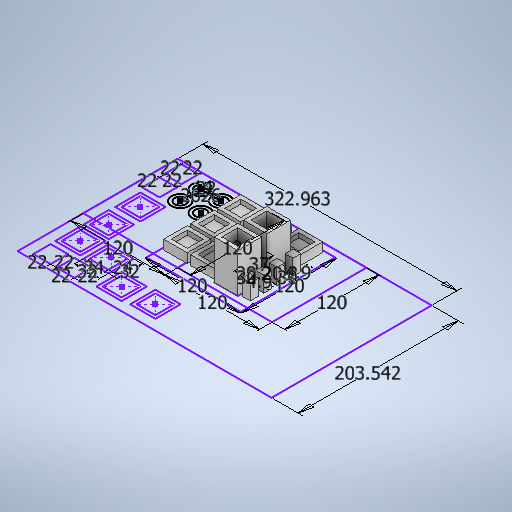
# Autodesk Inventor part: axie1
Saved by Autodesk Inventor 2025.1 (Build 291241000, 241)
## iProperties
Created: 2024-10-25
Part Number: axie1
Material: 一般
Document SubType Name: Modeling
Designer: youtian
Density: 1 g/cm^3
Appearance: 預設
Author: youtian
Autodesk Inventor part; units mm, degrees
ref_plane "YZ Plane" through (0, 0, 0) normal (1, 0, 0) x (0, 1, 0)
ref_plane "XZ Plane" through (0, 0, 0) normal (0, 1, 0) x (-1, 0, 0)
ref_plane "XY Plane" through (0, 0, 0) normal (0, 0, 1) x (1, 0, 0)
sketch "草圖1" plane through (0, 0, 0) normal (0, 1, 0) x (-1, 0, 0)
  circle A0 centre (0, 0) radius 7
  circle A1 centre (0, 0) radius 11
  line L0 (0, 0) -> (-26.517, 0)
  line L1 (0, 0) -> (0, 28.4195)
  circle A2 centre (-26, 0) radius 7
  circle A3 centre (-26, 0) radius 11
  circle A4 centre (0, 26) radius 7
  circle A5 centre (0, 26) radius 11
  circle A6 centre (-26, 26) radius 7
  circle A7 centre (-26, 26) radius 11
  dimension "d0" = 14
  dimension "d1" = 22
  dimension "d6" = 26
  dimension "d9" = 26
  constraints: 8 centre point, 5 coincident, 4 end point, 2 horizontal, 2 vertical, 12 other
  measures "d0" diameter of A0
  measures "d1" diameter of A1
  measures "d6" distance of A0.centre A2.centre
  measures "d9" distance of A0.centre A4.centre
sketch "草圖2" plane through (0, 0, 0) normal (0, 1, 0) x (-1, 0, 0)
  line L0 (-43.4184, -7.5692) -> (-73.4184, -7.5692)
  line L1 (-73.4184, -7.5692) -> (-73.4184, 22.4308)
  line L2 (-73.4184, 22.4308) -> (-43.4184, 22.4308)
  line L3 (-43.4184, 22.4308) -> (-43.4184, -7.5692)
  point P0 (0, 0)
  dimension "d14" = 30
  dimension "d15" = 30
  constraints: 8 end point, 2 parallel, 1 horizontal, 1 perpendicular
  measures "d14" distance of L1.end L2.end
  measures "d15" distance of L0.end L1.end
extrude "擠出3" add sketch "草圖2" along normal blind 12
sketch "草圖3" plane through (0, 12, 0) normal (0, 1, 0) x (1, 0, 0)
  line L0 (73.4184, -22.4308) -> (73.4184, 7.5692) projected
  line L1 (73.4184, 7.5692) -> (41.0142, -24.4308)
  line L2 (73.4184, 7.5692) -> (43.4184, 7.5692) projected
  line L3 (43.4184, 7.5692) -> (73.4184, -22.4308)
  line L4 (48.3184, 2.6692) -> (68.5184, 2.6692)
  line L5 (68.5184, 2.6692) -> (68.5184, -17.5308)
  line L6 (68.5184, -17.5308) -> (48.3184, -17.5308)
  line L7 (48.3184, -17.5308) -> (48.3184, 2.6692)
  line L8 (48.3184, 2.6692) -> (68.5184, -17.5308) construction
  line L9 (68.5184, 2.6692) -> (48.3184, -17.5308) construction
  point P0 (0, 0)
  point P1 (58.4184, -7.4308)
  dimension "d18" = 20.2
  dimension "d19" = 20.2
  constraints: 16 end point, 3 midpoint, 2 parallel, 1 horizontal, 1 perpendicular
  measures "d18" distance of L5.end L6.end
  measures "d19" distance of L4.end L5.end
extrude "擠出4" cut sketch "草圖3" against normal blind 5.6 contours L6 L7 L1 L3 | L3 L1 L4 L5 | L1 L3 L4 | L1 L7 L3
pattern_linear "矩形陣列1" count 2 spacing 34 along (1, 0, 0) count 3 spacing 34 along (0, 0, 1) of "擠出3", "擠出4"
sketch "草圖6" plane through (0, 0, 0) normal (0, 1, 0) x (-1, 0, 0)
  point P0 (0, 0)
sketch "草圖9" plane through (0, 0, 0) normal (0, 1, 0) x (-1, 0, 0)
  line L0 (-111.1142, 26.8484) -> (-141.1142, 26.8484)
  line L1 (-141.1142, 26.8484) -> (-141.1142, 56.8484)
  line L2 (-141.1142, 56.8484) -> (-111.1142, 56.8484)
  line L3 (-111.1142, 56.8484) -> (-111.1142, 26.8484)
  line L4 (-116.0142, 31.7484) -> (-136.2142, 31.7484)
  line L5 (-136.2142, 31.7484) -> (-136.2142, 51.9484)
  line L6 (-136.2142, 51.9484) -> (-116.0142, 51.9484)
  line L7 (-116.0142, 51.9484) -> (-116.0142, 31.7484)
  line L8 (-116.0142, 31.7484) -> (-136.2142, 51.9484) construction
  line L9 (-136.2142, 31.7484) -> (-116.0142, 51.9484) construction
  line L10 (-111.1142, 63.8484) -> (-141.1142, 63.8484)
  line L11 (-141.1142, 63.8484) -> (-141.1142, 93.8484)
  line L12 (-141.1142, 93.8484) -> (-111.1142, 93.8484)
  line L13 (-111.1142, 93.8484) -> (-111.1142, 63.8484)
  line L14 (-116.0142, 68.7484) -> (-136.2142, 68.7484)
  line L15 (-136.2142, 68.7484) -> (-136.2142, 88.9484)
  line L16 (-136.2142, 88.9484) -> (-116.0142, 88.9484)
  line L17 (-116.0142, 88.9484) -> (-116.0142, 68.7484)
  line L18 (-116.0142, 68.7484) -> (-136.2142, 88.9484) construction
  line L19 (-136.2142, 68.7484) -> (-116.0142, 88.9484) construction
  line L20 (-1.9445, 119.2719) -> (-33.9445, 119.2719)
  line L21 (-33.9445, 119.2719) -> (-33.9445, 151.2719)
  line L22 (-33.9445, 151.2719) -> (-1.9445, 151.2719)
  line L23 (-1.9445, 151.2719) -> (-1.9445, 119.2719)
  line L24 (-5.9445, 123.2719) -> (-29.9445, 123.2719)
  line L25 (-29.9445, 123.2719) -> (-29.9445, 147.2719)
  line L26 (-29.9445, 147.2719) -> (-5.9445, 147.2719)
  line L27 (-5.9445, 147.2719) -> (-5.9445, 123.2719)
  line L28 (-5.9445, 119.5982) -> (-29.9445, 143.5982) construction
  line L29 (-29.9445, 119.5982) -> (-5.9445, 143.5982) construction
  line L30 (35.5473, 81.3984) -> (3.5473, 81.3984)
  line L31 (3.5473, 81.3984) -> (3.5473, 113.3984)
  line L32 (3.5473, 113.3984) -> (35.5473, 113.3984)
  line L33 (35.5473, 113.3984) -> (35.5473, 81.3984)
  line L34 (31.5472, 85.3984) -> (7.5472, 85.3984)
  line L35 (7.5472, 85.3984) -> (7.5472, 109.3984)
  line L36 (7.5472, 109.3984) -> (31.5472, 109.3984)
  line L37 (31.5472, 109.3984) -> (31.5472, 85.3984)
  line L38 (31.5472, 85.3984) -> (7.5472, 109.3984) construction
  line L39 (7.5472, 85.3984) -> (31.5472, 109.3984) construction
  line L40 (34.8593, 41.843) -> (2.8593, 41.843)
  line L41 (30.8593, 45.843) -> (6.8593, 45.843)
  line L42 (6.8593, 45.843) -> (6.8593, 69.843)
  line L43 (2.8593, 41.843) -> (2.8593, 73.843)
  line L44 (6.8593, 69.843) -> (30.8593, 69.843)
  line L45 (30.8593, 45.843) -> (6.8593, 69.843) construction
  line L46 (6.8593, 45.843) -> (30.8593, 69.843) construction
  line L47 (2.8593, 73.843) -> (34.8593, 73.843)
  line L48 (30.8593, 69.843) -> (30.8593, 45.843)
  line L49 (34.8593, 73.843) -> (34.8593, 41.843)
  line L50 (35.5473, 117.4293) -> (3.5473, 117.4293)
  line L51 (31.5472, 121.4294) -> (7.5472, 121.4294)
  line L52 (7.5472, 121.4294) -> (7.5472, 145.4294)
  line L53 (3.5473, 117.4293) -> (3.5473, 149.4293)
  line L54 (7.5472, 145.4294) -> (31.5472, 145.4294)
  line L55 (31.5472, 121.4294) -> (7.5472, 145.4294) construction
  line L56 (7.5472, 121.4294) -> (31.5472, 145.4294) construction
  line L57 (3.5473, 149.4293) -> (35.5473, 149.4293)
  line L58 (31.5472, 145.4294) -> (31.5472, 121.4294)
  line L59 (35.5473, 149.4293) -> (35.5473, 117.4293)
  line L60 (-40.805, 141.4327) -> (-72.805, 141.4327)
  line L61 (-44.805, 145.4328) -> (-68.805, 145.4328)
  line L62 (-68.805, 145.4328) -> (-68.805, 169.4328)
  line L63 (-72.805, 141.4327) -> (-72.805, 173.4327)
  line L64 (-68.805, 169.4328) -> (-44.805, 169.4328)
  line L65 (-44.805, 145.4328) -> (-68.805, 169.4328) construction
  line L66 (-68.805, 145.4328) -> (-44.805, 169.4328) construction
  line L67 (-72.805, 173.4327) -> (-40.805, 173.4327)
  line L68 (-44.805, 169.4328) -> (-44.805, 145.4328)
  line L69 (-40.805, 173.4327) -> (-40.805, 141.4327)
  line L70 (-81.8163, 139.4435) -> (-113.8163, 139.4435)
  line L71 (-85.8164, 143.4436) -> (-109.8164, 143.4436)
  line L72 (-109.8164, 143.4436) -> (-109.8164, 167.4436)
  line L73 (-113.8163, 139.4435) -> (-113.8163, 171.4435)
  line L74 (-109.8164, 167.4436) -> (-85.8164, 167.4436)
  line L75 (-85.8164, 143.4436) -> (-109.8164, 167.4436) construction
  line L76 (-109.8164, 143.4436) -> (-85.8164, 167.4436) construction
  line L77 (-113.8163, 171.4435) -> (-81.8163, 171.4435)
  line L78 (-85.8164, 167.4436) -> (-85.8164, 143.4436)
  line L79 (-81.8163, 171.4435) -> (-81.8163, 139.4435)
  point P0 (0, 0)
  point P1 (-126.1142, 41.8484)
  point P2 (-126.1142, 78.8484)
  point P3 (-17.9445, 131.5982)
  point P4 (19.5472, 97.3984)
  point P5 (18.8593, 57.843)
  point P6 (19.5472, 133.4294)
  point P7 (-56.805, 157.4328)
  point P8 (-97.8164, 155.4436)
  dimension "d73" = 50.747
  dimension "d54" = 30
  dimension "d55" = 30
  dimension "d56" = 20.2
  dimension "d57" = 20.2
  dimension "d60" = 37
  dimension "d69" = 32
  dimension "d70" = 32
  dimension "d71" = 24
  dimension "d72" = 24
  dimension "d141" = 4.9
  dimension "d142" = 4.9
  constraints: 160 end point, 8 parallel, 4 horizontal, 4 midpoint, 4 perpendicular, 2 vertical, 1 collinear, 18 other
  measures "d54" distance of L1.end L2.end
  measures "d55" distance of L0.end L1.end
  measures "d56" distance of L5.end L6.end
  measures "d57" distance of L4.end L5.end
  measures "d60" distance of L0.start L10.start
  measures "d69" distance of L22.start L22.end
  measures "d70" distance of L20.end L22.start
  measures "d71" distance of L26.start L26.end
  measures "d72" distance of L24.end L26.start
  measures "d141" horizontal distance of L0.end L4.end
  measures "d142" horizontal distance of L5.end L1.end
extrude "擠出9" add sketch "草圖9" along normal blind 50 contours L0 L1 L2 L3 | L10 L11 L12 L13
sketch "草圖10" plane through (0, 0, 0) normal (0, 1, 0) x (-1, 0, 0)
  line L0 (48.2716, 184.5725) -> (-274.6912, 184.5725)
  line L1 (-274.6912, 184.5725) -> (-274.6912, -18.9692)
  line L2 (-274.6912, -18.9692) -> (48.2716, -18.9692)
  line L3 (48.2716, -18.9692) -> (48.2716, 184.5725)
  line L4 (48.2716, -18.9692) -> (-71.7284, -18.9692)
  line L5 (-71.7284, -18.9692) -> (-71.7284, 101.0308)
  line L6 (-71.7284, 101.0308) -> (48.2716, 101.0308)
  line L7 (48.2716, 101.0308) -> (48.2716, -18.9692)
  line L8 (-71.7284, -18.9692) -> (-191.7284, -18.9692)
  line L9 (-191.7284, -18.9692) -> (-191.7284, 101.0308)
  line L10 (-191.7284, 101.0308) -> (-71.7284, 101.0308)
  line L11 (-71.7284, 101.0308) -> (-71.7284, -18.9692)
  point P0 (0, 0)
  dimension "d99" = 322.9628
  dimension "d100" = 203.5417
  dimension "d135" = 120
  dimension "d136" = 120
  dimension "d137" = 120
  dimension "d138" = 120
  constraints: 24 end point, 6 parallel, 3 horizontal, 3 perpendicular
  measures "d99" distance of L1.end L2.end
  measures "d100" distance of L0.end L1.end
  measures "d135" distance of L5.end L6.end
  measures "d136" distance of L4.end L5.end
  measures "d137" distance of L9.end L10.end
  measures "d138" distance of L8.end L9.end
sketch "草圖11" plane through (0, 0, 0) normal (0, 1, 0) x (-1, 0, 0)
  line L0 (35.0654, 155.7952) -> (13.0654, 155.7952)
  line L1 (13.0654, 155.7952) -> (13.0654, 177.7952)
  line L2 (13.0654, 177.7952) -> (35.0654, 177.7952)
  line L3 (35.0654, 177.7952) -> (35.0654, 155.7952)
  line L4 (4.7905, 155.7952) -> (-17.2095, 155.7952)
  line L5 (-17.2095, 155.7952) -> (-17.2095, 177.7952)
  line L6 (-17.2095, 177.7952) -> (4.7905, 177.7952)
  line L7 (4.7905, 177.7952) -> (4.7905, 155.7952)
  point P0 (0, 0)
  dimension "d101" = 22
  dimension "d102" = 22
  dimension "d103" = 22
  dimension "d104" = 22
  constraints: 16 end point, 4 parallel, 2 horizontal, 2 perpendicular
  measures "d101" distance of L1.end L2.end
  measures "d102" distance of L0.end L1.end
  measures "d103" distance of L5.end L6.end
  measures "d104" distance of L4.end L5.end
sketch "草圖12" plane through (0, 0, 0) normal (0, 1, 0) x (-1, 0, 0)
  line L0 (17.1987, 35.1037) -> (39.1987, 35.1037)
  line L1 (39.1987, 35.1037) -> (39.1987, 13.1037)
  line L2 (39.1987, 13.1037) -> (17.1987, 13.1037)
  line L3 (17.1987, 13.1037) -> (17.1987, 35.1037)
  line L4 (17.9153, 6.7257) -> (39.9153, 6.7257)
  line L5 (39.9153, 6.7257) -> (39.9153, -15.2743)
  line L6 (39.9153, -15.2743) -> (17.9153, -15.2743)
  line L7 (17.9153, -15.2743) -> (17.9153, 6.7257)
  point P0 (0, 0)
  dimension "d105" = 22
  dimension "d106" = 22
  dimension "d107" = 22
  dimension "d108" = 22
  constraints: 16 end point, 4 parallel, 2 horizontal, 2 perpendicular
  measures "d105" distance of L1.end L2.end
  measures "d106" distance of L0.end L1.end
  measures "d107" distance of L5.end L6.end
  measures "d108" distance of L4.end L5.end
sketch "草圖14" plane through (0, 0, 0) normal (0, 1, 0) x (-1, 0, 0)
  line L0 (-154.5089, 57.5113) -> (-154.5089, 47.5113)
  line L1 (-154.5089, 47.5113) -> (-144.5089, 47.5113)
  line L2 (-144.5089, 47.5113) -> (-144.5089, 57.5113)
  line L3 (-144.5089, 57.5113) -> (-154.5089, 57.5113)
  line L4 (-154.5089, 27.2143) -> (-154.5089, 37.2143)
  line L5 (-154.5089, 37.2143) -> (-144.5089, 37.2143)
  line L6 (-144.5089, 37.2143) -> (-144.5089, 27.2143)
  line L7 (-144.5089, 27.2143) -> (-154.5089, 27.2143)
  line L8 (-154.5089, 91.4866) -> (-154.5089, 81.4866)
  line L9 (-154.5089, 81.4866) -> (-144.5089, 81.4866)
  line L10 (-144.5089, 81.4866) -> (-144.5089, 91.4866)
  line L11 (-144.5089, 91.4866) -> (-154.5089, 91.4866)
  line L12 (-154.5089, 64.3577) -> (-154.5089, 74.3577)
  line L13 (-154.5089, 74.3577) -> (-144.5089, 74.3577)
  line L14 (-144.5089, 74.3577) -> (-144.5089, 64.3577)
  line L15 (-144.5089, 64.3577) -> (-154.5089, 64.3577)
  point P0 (0, 0)
  dimension "d123" = 10
  dimension "d124" = 10
  dimension "d125" = 10
  dimension "d126" = 10
  dimension "d143" = 10
  dimension "d144" = 10
  dimension "d145" = 10
  dimension "d146" = 10
  constraints: 32 end point, 8 parallel, 4 perpendicular, 1 point on line
  measures "d123" distance of L2.end L1.end
  measures "d124" distance of L1.end L0.end
  measures "d125" distance of L5.end L6.end
  measures "d126" distance of L4.end L5.end
  measures "d143" distance of L10.end L9.end
  measures "d144" distance of L9.end L8.end
  measures "d145" distance of L13.end L14.end
  measures "d146" distance of L12.end L13.end
extrude "擠出14" add sketch "草圖14" along normal blind 20
pattern_linear "矩形陣列5" count 2 spacing 74 along (1, 0, 0) of "擠出3", "擠出4"
sketch "草圖15" plane through (0, 0, 0) normal (0, 1, 0) x (-1, 0, 0)
  line L0 (-141.1142, 56.8484) -> (-141.1142, 26.8484) projected
  line L1 (-40.5554, -10.4383) -> (-160.5554, -10.4383)
  line L2 (-160.5554, -10.4383) -> (-160.5554, 109.5617)
  line L3 (-160.5554, 109.5617) -> (-40.5554, 109.5617)
  line L4 (-40.5554, 109.5617) -> (-40.5554, -10.4383)
  point P0 (0, 0)
  dimension "d139" = 120
  dimension "d140" = 120
  constraints: 8 end point, 2 parallel, 1 horizontal, 1 perpendicular
  measures "d139" distance of L2.end L3.end
  measures "d140" distance of L1.end L2.end
